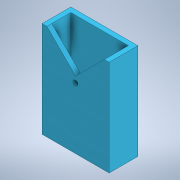
# Autodesk Inventor part: ENGR131 KC Design
Saved by Autodesk Inventor 2020 (Build 240168000, 168)
## iProperties
Created: 2019-11-06
Part Number: ENGR131 KC Design
Material: Concrete Masonry Units
Document SubType Name: Modeling
Designer: camde
Density: 2.40731 g/cm^3
Appearance: Turquoise
Mass: 463.099 g
Surface Area: 614.234 cm^2
Volume: 192.372 cm^3
Author: camde
Autodesk Inventor part; units mm, degrees
ref_plane "YZ Plane" through (0, 0, 0) normal (1, 0, 0) x (0, 1, 0)
ref_plane "XZ Plane" through (0, 0, 0) normal (0, 1, 0) x (-1, 0, 0)
ref_plane "XY Plane" through (0, 0, 0) normal (0, 0, 1) x (1, 0, 0)
sketch "Sketch1" plane through (0, 0, 0) normal (0, 0, 1) x (1, 0, 0)
  line L0 (-12.1245, 12.5373) -> (64.0755, 12.5373)
  line L1 (64.0755, 12.5373) -> (64.0755, -114.4627)
  line L2 (64.0755, -114.4627) -> (-12.1245, -114.4627)
  line L3 (-12.1245, -114.4627) -> (-12.1245, 12.5373)
  point P0 (0, 0)
  dimension "d0" = 76.2
  dimension "d1" = 127
  constraints: 8 end point, 2 parallel, 1 horizontal, 1 perpendicular
  measures "d0" distance of L1.end L2.end
  measures "d1" distance of L0.end L1.end
extrude "Extrusion1" add sketch "Sketch1" along normal blind 6.35
sketch "Sketch2" plane through (0, 0, 6.35) normal (0, 0, 1) x (1, 0, 0)
  line L0 (-12.1245, -114.4627) -> (64.0755, -114.4627) projected
  line L1 (25.9755, -114.4627) -> (25.9755, 12.062) construction
  line L2 (21.4802, -114.4627) -> (21.4802, -38.2627)
  line L3 (30.4708, -114.4627) -> (30.4708, -38.2627)
  line L4 (21.4802, -38.2627) -> (30.4708, -38.2627)
  line L5 (21.4802, -114.4627) -> (30.4708, -114.4627)
  point P0 (0, 0)
  dimension "d4" = 76.2
  constraints: 10 end point, 2 horizontal, 2 symmetric about line, 2 vertical, 1 midpoint, 1 point on line
  measures "d4" distance of L2.start L2.end
extrude "Extrusion2" add sketch "Sketch2" along normal blind 25.4
sketch "Sketch3" plane through (0, 0, 31.75) normal (0, 0, 1) x (1, 0, 0)
  line L0 (64.0755, -114.4627) -> (64.0755, 12.5373) projected
  line L1 (-12.1245, -114.4627) -> (64.0755, -114.4627)
  line L2 (64.0755, -114.4627) -> (64.0755, 0)
  line L3 (64.0755, 0) -> (-12.1245, 0)
  line L4 (-12.1245, 0) -> (-12.1245, -114.4627)
  point P0 (0, 0)
  constraints: 8 end point, 2 parallel, 1 horizontal, 1 perpendicular, 1 point on line
extrude "Extrusion3" add sketch "Sketch3" along normal blind 6.35
sketch "Sketch4" plane through (0, 0, 31.75) normal (0, 0, -1) x (-1, 0, 0)
  point P0 (0, 0)
sketch "Sketch5" plane through (0, 0, 6.35) normal (0, 0, 1) x (1, 0, 0)
  line L0 (21.4802, -38.2627) -> (30.4708, -38.2627) projected
  line L1 (25.9755, -38.2627) -> (25.9755, -33.1827) construction
  circle A0 centre (25.9755, -33.1827) radius 3.175
  point P0 (0, 0)
  dimension "d9" = 5.08
  dimension "d10" = 6.35
  constraints: 2 end point, 1 centre point, 1 coincident, 1 midpoint, 1 vertical
  measures "d9" distance of L1.start L1.end
  measures "d10" diameter of A0
extrude "Extrusion4" cut sketch "Sketch5" along normal mid plane 76.2
sketch "Sketch6" plane through (64.0755, -114.4627, 31.75) normal (1, 0, 0) x (0, 0, -1)
  line L0 (31.75, 127) -> (31.75, 0) projected
  line L1 (-6.35, 114.4627) -> (31.75, 114.4627)
  line L2 (31.75, 114.4627) -> (31.75, 0)
  line L3 (31.75, 0) -> (-6.35, 0)
  line L4 (-6.35, 0) -> (-6.35, 114.4627)
  constraints: 8 end point, 2 parallel, 1 horizontal, 1 perpendicular
extrude "Extrusion5" add sketch "Sketch6" along normal blind 6.35
sketch "Sketch7" plane through (-12.1245, -114.4627, 31.75) normal (-1, 0, 0) x (0, 0, 1)
  line L0 (0, 114.4627) -> (6.35, 114.4627) projected
  line L1 (-31.75, 0) -> (-25.4, 0) projected
  line L2 (6.35, 114.4627) -> (-31.75, 114.4627)
  line L3 (-31.75, 114.4627) -> (-31.75, 0)
  line L4 (-31.75, 0) -> (6.35, 0)
  line L5 (6.35, 0) -> (6.35, 114.4627)
  constraints: 8 end point, 2 parallel, 1 horizontal, 1 perpendicular
extrude "Extrusion6" add sketch "Sketch7" along normal blind 6.35
sketch "Sketch8" plane through (64.0755, 0, 31.75) normal (0, 1, 0) x (1, 0, 0)
  line L0 (-82.55, 31.75) -> (6.35, 31.75) projected
  line L1 (0, 0) -> (-76.2, 0) projected
  line L2 (-82.55, 31.75) -> (-76.2, 31.75)
  line L3 (-76.2, 31.75) -> (-76.2, 0)
  line L4 (-82.55, 0) -> (-82.55, 31.75)
  line L5 (6.35, 31.75) -> (6.35, -6.35) projected
  line L6 (-76.2, 0) -> (0, 0)
  line L7 (6.35, 0) -> (6.35, -6.35)
  line L8 (6.35, -6.35) -> (-82.55, -6.35)
  line L9 (-82.55, -6.35) -> (-82.55, 0)
  line L10 (0, 31.75) -> (0, 25.4) projected
  line L11 (0, 0) -> (0, 31.75)
  line L12 (0, 31.75) -> (6.35, 31.75)
  line L13 (6.35, 31.75) -> (6.35, 0)
  point P0 (-64.0755, 31.75)
  constraints: 20 end point, 4 parallel, 2 horizontal, 2 perpendicular, 1 point on line
extrude "Extrusion7" add sketch "Sketch8" along normal blind 12.7 contours L0 L3 L1 L11 L10 L5 L8 L9 L4
sketch "Sketch9" plane through (64.0755, 12.5373, 6.35) normal (0, 1, 0) x (1, 0, 0)
  line L0 (-76.2, 0) -> (-42.5953, 0) projected
  line L1 (-82.55, 6.35) -> (6.35, 6.35) projected
  line L2 (-76.2, 0) -> (0.0054, 0)
  line L3 (0.0054, 0) -> (0.0054, 6.35)
  line L4 (0.0054, 6.35) -> (-76.2, 6.35)
  line L5 (-76.2, 6.35) -> (-76.2, 0)
  point P0 (-64.0755, 6.35)
  constraints: 8 end point, 2 parallel, 1 horizontal, 1 perpendicular, 1 point on line
extrude "Extrusion8" add sketch "Sketch9" along normal up to surface (0.1627 mm away)
sketch "Sketch10" plane through (0, 0, 38.1) normal (0, 0, 1) x (1, 0, 0)
  line L0 (64.0755, 12.7) -> (-12.1245, 12.7) construction
  line L1 (64.0755, -114.4627) -> (64.0755, 12.7) projected
  line L2 (-12.1245, 12.7) -> (64.0755, 12.7) construction
  line L3 (64.0755, 12.7) -> (64.0755, -63.5) construction
  line L4 (64.0755, -63.5) -> (-12.1245, -63.5) construction
  line L5 (-12.1245, -63.5) -> (-12.1245, 12.7) construction
  line L6 (-12.1245, 12.7) -> (25.9755, -25.4)
  line L7 (64.0755, 12.7) -> (25.9755, -25.4)
  line L8 (-12.1245, -114.4627) -> (-12.1245, 12.7) projected
  line L9 (-12.1245, 12.7) -> (64.0755, 12.7)
  point P0 (0, 0)
  dimension "d21" = 76.2
  constraints: 14 end point, 2 parallel, 2 perpendicular, 1 horizontal, 1 point on line
  measures "d21" distance of L2.end L3.end
extrude "Extrusion9" cut sketch "Sketch10" against normal blind 25.4
body "Solid1"
